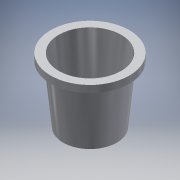
# Autodesk Inventor part: Bucket
Saved by Autodesk Inventor 2018 (Build 220112000, 112)
## iProperties
Created: 2017-10-26
Part Number: Bucket
Material: LCP Plastic
Document SubType Name: Modeling
Designer: kurtis
Density: 1.626 g/cm^3
Appearance: Smooth - White
Author: kurtis
Autodesk Inventor part; units mm, degrees
ref_plane "YZ Plane" through (0, 0, 0) normal (1, 0, 0) x (0, 1, 0)
ref_plane "XZ Plane" through (0, 0, 0) normal (0, 1, 0) x (-1, 0, 0)
ref_plane "XY Plane" through (0, 0, 0) normal (0, 0, 1) x (1, 0, 0)
sketch "Sketch1" plane through (0, 0, 0) normal (0, 0, 1) x (1, 0, 0)
  spline S0 degree 3 poles (-35.9347, -28.034) (-38.2518, -14.064) (-40.2964, 0.4145) (-42.8197, 25.9903) (-43.5988, 38.0212) (-43.5918, 49.563) knots -7.717139 -7.717139 -7.717139 -7.717139 -3.462559 -3.462559 0 0 0 0 construction
  line L0 (-43.5918, 49.563) -> (-41.8107, 49.563) construction
  line L1 (-41.8107, 49.563) -> (-41.8107, 49.562) construction
  spline S1 degree 3 poles (-41.8107, 49.562) (-41.8177, 37.9419) (-41.0223, 25.8121) (-38.4526, 0.0021) (-36.3657, -14.6475) (-34.005, -28.7707) knots -7.776786 -7.776786 -7.776786 -7.776786 -4.295739 -4.295739 0 0 0 0 construction
  spline S2 degree 3 poles (-34.005, -28.7707) (-29.7185, -31.4849) (-25.241, -33.8415) (-16.726, -37.4394) (-12.7722, -38.7952) (-7.5781, -40.171) (-6.3496, -40.4679) (-4.3584, -40.8946) (-3.5445, -41.0548) (-2.2442, -41.2757) (-1.7048, -41.3577) (-0.5553, -41.4951) (0.0791, -41.5458) (1.412, -41.5512) (2.0749, -41.5002) (3.2552, -41.3599) (3.7943, -41.2781) (4.6855, -41.1272) (5.068, -41.0573) (5.4504, -40.9834) knots -16.028143 -16.028143 -16.028143 -16.028143 -11.719555 -11.719555 -8.174537 -8.174537 -7.104934 -7.104934 -6.414126 -6.414126 -5.960259 -5.960259 -5.415102 -5.415102 -4.841155 -4.841155 -4.386079 -4.386079 -4.054178 -4.054178 -4.054178 -4.054178 construction
  line L2 (5.4504, -40.9834) -> (5.4504, -41.788) construction
  spline S3 degree 3 poles (5.4504, -41.788) (5.7804, -41.7248) (6.1108, -41.6585) (7.4816, -41.373) (8.542, -41.1266) (12.6773, -40.0825) (15.7697, -39.1153) (23.5096, -36.2333) (28.0566, -34.0916) (32.4276, -31.5847) knots -2.907205 -2.907205 -2.907205 -2.907205 -2.805503 -2.805503 -2.480194 -2.480194 -1.5117 -1.5117 -0.000033 -0.000033 -0.000033 -0.000033 construction
  line L3 (32.4276, -31.5847) -> (32.4276, -30.6767) construction
  spline S4 degree 3 poles (32.4276, -30.6767) (33.4861, -30.0628) (34.5339, -29.4273) (35.5709, -28.7707) knots -0.368225 -0.368225 -0.368225 -0.368225 0 0 0 0 construction
  spline S5 degree 3 poles (35.5709, -28.7707) (37.9317, -14.6472) (40.0186, 0.0026) (42.5883, 25.8126) (43.3836, 37.9422) (43.3766, 49.562) knots -7.787874 -7.787874 -7.787874 -7.787874 -3.485936 -3.485936 0 0 0 0 construction
  line L4 (43.3766, 49.562) -> (43.3766, 49.563) construction
  line L5 (43.3766, 49.563) -> (45.1577, 49.563)
  spline S6 degree 3 poles (45.1577, 49.563) (45.1647, 38.021) (44.3856, 25.9899) (41.8623, 0.4141) (39.8177, -14.0642) (37.5007, -28.034) knots -7.705654 -7.705654 -7.705654 -7.705654 -4.248191 -4.248191 0 0 0 0 construction
  line L6 (37.5007, -28.034) -> (48.5285, -28.034) construction
  line L7 (48.5285, -28.034) -> (48.5285, -36.162) construction
  line L8 (48.5285, -36.162) -> (46.7478, -36.162) construction
  line L9 (46.7478, -36.162) -> (46.7478, -29.812) construction
  line L10 (46.7478, -29.812) -> (37.2038, -29.812) construction
  spline S7 degree 3 poles (37.2038, -29.812) (35.6372, -30.8226) (34.0451, -31.7862) (32.4276, -32.7015) knots -11.950136 -11.950136 -11.950136 -11.950136 -10.890229 -10.890229 -10.890229 -10.890229 construction
  line L11 (32.4276, -32.7015) -> (32.4276, -32.0799) construction
  spline S8 degree 3 poles (32.4276, -32.0799) (27.095, -35.12) (21.5117, -37.6144) (13.3692, -40.2993) (10.9904, -40.9781) (7.7119, -41.7604) (6.7769, -41.9667) (5.7244, -42.1749) (5.588, -42.2014) (5.4504, -42.2277) knots -3.070497 -3.070497 -3.070497 -3.070497 -1.259015 -1.259015 -0.53243 -0.53243 -0.251343 -0.251343 -0.210092 -0.210092 -0.210092 -0.210092 construction
  line L12 (5.4504, -42.2277) -> (5.4504, -42.7803) construction
  spline S9 degree 3 poles (5.4504, -42.7803) (5.1069, -42.8454) (4.7641, -42.9072) (3.8999, -43.0532) (3.3486, -43.1369) (2.1677, -43.2787) (1.5091, -43.3322) (0.2091, -43.3372) (-0.4396, -43.2978) (-1.7714, -43.1385) (-2.3225, -43.055) (-3.6456, -42.8319) (-4.4712, -42.6709) (-8.7991, -41.7533) (-13.1529, -40.5742) (-24.2344, -36.3726) (-30.0905, -33.3906) (-35.6379, -29.812) knots -5.386233 -5.386233 -5.386233 -5.386233 -5.187344 -5.187344 -4.877187 -4.877187 -4.500213 -4.500213 -4.148864 -4.148864 -3.914531 -3.914531 -3.55984 -3.55984 -1.980467 -1.980467 0 0 0 0 construction
  line L13 (-35.6379, -29.812) -> (-45.1819, -29.812) construction
  line L14 (-45.1819, -29.812) -> (-45.1819, -36.162) construction
  line L15 (-45.1819, -36.162) -> (-46.9626, -36.162) construction
  line L16 (-46.9626, -36.162) -> (-46.9626, -28.034) construction
  line L17 (-46.9626, -28.034) -> (-35.9347, -28.034) construction
  line L18 (45.1577, 49.563) -> (46.9357, 49.563)
  line L19 (46.9357, 49.563) -> (46.9357, 43.213)
  line L20 (46.9357, 43.213) -> (49.4757, 43.213)
  line L21 (49.4757, 43.213) -> (49.4757, 52.103)
  line L22 (43.3766, 49.563) -> (41.5986, 49.563)
  line L23 (35.5709, -28.7707) -> (33.7929, -28.7707) construction
  line L24 (33.7929, -28.7707) -> (41.5986, 49.563)
  line L25 (41.5986, 49.563) -> (39.0586, 49.563) construction
  line L26 (33.7929, -28.7707) -> (31.2529, -28.7707) construction
  line L27 (33.7929, -28.7707) -> (0, -28.7707)
  line L28 (33.7929, -28.7707) -> (34.0448, -26.2432) construction
  line L29 (0, -28.7707) -> (0, -26.2307)
  line L30 (31.5048, -26.2307) -> (39.0586, 49.563)
  line L31 (31.5048, -26.2307) -> (0, -26.2307)
  line L32 (39.0586, 49.563) -> (39.3117, 52.103)
  line L33 (39.3117, 52.103) -> (49.4757, 52.103)
  point P0 (0, 0)
  dimension "d0" = 1.778
  dimension "d1" = 6.35
  dimension "d2" = 2.54
  dimension "d3" = 8.89
  dimension "d4" = 1.778
  dimension "d5" = 1.778
  dimension "d6" = 2.54
  dimension "d7" = 2.54
  dimension "d9" = 2.54
  dimension "d10" = 2.54
  dimension "d11" = 2.5287
  dimension "d12" = 95.691
  dimension "d13" = 95.692
  constraints: 68 end point, 14 horizontal, 8 vertical, 2 perpendicular, 1 point on line, 57 other
  measures "d0" distance of L5.end L18.end
  measures "d1" distance of L18.end L19.end
  measures "d2" distance of L19.end L20.end
  measures "d3" distance of L20.end L21.end
  measures "d4" distance of L4.end L22.end
  measures "d5" distance of L23.start L23.end
  measures "d6" distance of L22.end L25.end
  measures "d7" distance of L23.end L26.end
  measures "d9" distance of L27.end L29.end
  measures "d10" distance from line of L27 L30.start
  measures "d11" distance from line of L24 L30.start
  measures "d12" angle of L24 L27
  measures "d13" angle of L30 L31
revolve "Revolution1" add sketch "Sketch1" angle 360 about axis through (0, -28.7707, 0) along (0, 1, 0)
sketch "Sketch2" plane through (0, -26.2307, 0) normal (0, 1, 0) x (1, 0, 0)
  circle A0 centre (0, 0) radius 2.54
  line L0 (0, 0) -> (0, -31.5048) construction
  circle A1 centre (0, 0) radius 31.5048 construction
  circle A2 centre (0, -7.62) radius 2.54
  circle A3 centre (0, -15.24) radius 2.54
  circle A4 centre (0, -22.86) radius 2.54
  circle A5 centre (0, 7.62) radius 2.54
  circle A6 centre (0, 0) radius 2.54
  circle A7 centre (0, -7.62) radius 2.54
  circle A8 centre (0, -15.24) radius 2.54
  circle A9 centre (0, 15.24) radius 2.54
  circle A10 centre (0, 7.62) radius 2.54
  circle A11 centre (0, 0) radius 2.54
  circle A12 centre (0, -7.62) radius 2.54
  circle A13 centre (0, 22.86) radius 2.54
  circle A14 centre (0, 15.24) radius 2.54
  circle A15 centre (0, 7.62) radius 2.54
  circle A16 centre (0, 0) radius 2.54
  line L1 (0, 0) -> (-15.3445, 0) construction
  circle A17 centre (16.1645, -16.1645) radius 2.54
  circle A18 centre (10.7763, -10.7763) radius 2.54
  circle A19 centre (5.3882, -5.3882) radius 2.54
  circle A20 centre (0, 0) radius 2.54
  circle A21 centre (-5.3882, 5.3882) radius 2.54
  circle A22 centre (-10.7763, 10.7763) radius 2.54
  circle A23 centre (-16.1645, 16.1645) radius 2.54
  circle A24 centre (22.86, 0) radius 2.54
  circle A25 centre (15.24, 0) radius 2.54
  circle A26 centre (7.62, 0) radius 2.54
  circle A27 centre (0, 0) radius 2.54
  circle A28 centre (-7.62, 0) radius 2.54
  circle A29 centre (-15.24, 0) radius 2.54
  circle A30 centre (-22.86, 0) radius 2.54
  circle A31 centre (16.1645, 16.1645) radius 2.54
  circle A32 centre (10.7763, 10.7763) radius 2.54
  circle A33 centre (5.3882, 5.3882) radius 2.54
  circle A34 centre (0, 0) radius 2.54
  circle A35 centre (-5.3882, -5.3882) radius 2.54
  circle A36 centre (-10.7763, -10.7763) radius 2.54
  circle A37 centre (-16.1645, -16.1645) radius 2.54
  circle A38 centre (0, 22.86) radius 2.54
  circle A39 centre (0, 15.24) radius 2.54
  circle A40 centre (0, 7.62) radius 2.54
  circle A41 centre (0, 0) radius 2.54
  circle A42 centre (0, -7.62) radius 2.54
  circle A43 centre (0, -15.24) radius 2.54
  circle A44 centre (0, -22.86) radius 2.54
  circle A45 centre (-16.1645, 16.1645) radius 2.54
  circle A46 centre (-10.7763, 10.7763) radius 2.54
  circle A47 centre (-5.3882, 5.3882) radius 2.54
  circle A48 centre (0, 0) radius 2.54
  circle A49 centre (5.3882, -5.3882) radius 2.54
  circle A50 centre (10.7763, -10.7763) radius 2.54
  circle A51 centre (16.1645, -16.1645) radius 2.54
  circle A52 centre (-22.86, 0) radius 2.54
  circle A53 centre (-15.24, 0) radius 2.54
  circle A54 centre (-7.62, 0) radius 2.54
  circle A55 centre (0, 0) radius 2.54
  circle A56 centre (7.62, 0) radius 2.54
  circle A57 centre (15.24, 0) radius 2.54
  circle A58 centre (22.86, 0) radius 2.54
  circle A59 centre (-16.1645, -16.1645) radius 2.54
  circle A60 centre (-10.7763, -10.7763) radius 2.54
  circle A61 centre (-5.3882, -5.3882) radius 2.54
  circle A62 centre (0, 0) radius 2.54
  circle A63 centre (5.3882, 5.3882) radius 2.54
  circle A64 centre (10.7763, 10.7763) radius 2.54
  circle A65 centre (16.1645, 16.1645) radius 2.54
  dimension "d15" = 5.08
  dimension "d18" = 7.62
  dimension "d21" = 7.62
  dimension "d26" = 360
  constraints: 65 centre point, 4 end point, 3 vertical, 1 coincident, 1 horizontal, 1 vertical alignment, 144 other
  measures "d15" diameter of A0
  measures "d18" distance of L0.start A2.centre
  measures "d21" distance of L0.start A5.centre
extrude "Extrusion1" cut sketch "Sketch2" against normal blind 49.2125
equation "\"d4\" = d0"
equation "\"d5\" = d0"
body "Solid1"
